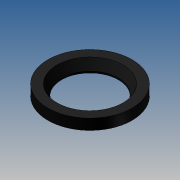
# Autodesk Inventor part: unutrasnja plastika
Saved by Autodesk Inventor 2014 (Build 180170000, 170)
## iProperties
Created: 2011-11-30
Part Number: unutrasnja plastika
Material: Generic
Document SubType Name: Modeling
Designer: slazh bliskovic
Density: 1 g/cm^3
Mass: 0.301933 g
Surface Area: 4.94917 cm^2
Volume: 0.301933 cm^3
Appearance: Glossy - Black
Author: slazh bliskovic
Autodesk Inventor part; units mm, degrees
ref_plane "YZ Plane" through (0, 0, 0) normal (1, 0, 0) x (0, 1, 0)
ref_plane "XZ Plane" through (0, 0, 0) normal (0, 1, 0) x (-1, 0, 0)
ref_plane "XY Plane" through (0, 0, 0) normal (0, 0, 1) x (1, 0, 0)
sketch "Sketch1" plane through (0, 0, 0) normal (0, 0, 1) x (1, 0, 0)
  circle A0 centre (24.0765, 0.0001) radius 9.25 projected
  circle A1 centre (24.0765, 0.0001) radius 6.25
  point P0 (0, 0)
  dimension "d0" = 12.5
  constraints: 1 centre point, 1 coincident
  measures "d0" diameter of A1
extrude "Extrusion1" add sketch "Sketch1" along normal blind 2.35
chamfer "Chamfer1" distance 1 distance2 2 1 edges at (17.8265, 0.0001, 2.35) measured on face at (32.2369, -0.7378, 2.35)
body "Solid1"
